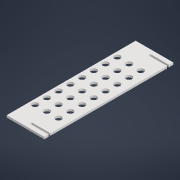
# Autodesk Inventor part: ChromoHolder
Saved by Autodesk Inventor 2021.3 (Build 253353000, 353)
## iProperties
Created: 2019-07-01
Part Number: ChromoHolder
Material: Generic
Document SubType Name: Modeling
Designer: eugen
Density: 1 g/cm^3
Appearance: Default
Author: eugen
Autodesk Inventor part; units mm, degrees
ref_plane "YZ Plane" through (0, 0, 0) normal (1, 0, 0) x (0, 1, 0)
ref_plane "XZ Plane" through (0, 0, 0) normal (0, 1, 0) x (-1, 0, 0)
ref_plane "XY Plane" through (0, 0, 0) normal (0, 0, 1) x (1, 0, 0)
sketch "Sketch1" plane through (0, 0, 0) normal (0, 1, 0) x (-1, 0, 0)
  line L0 (0, 0) -> (100.203, 0)
  line L1 (100.203, 0) -> (100.203, -387.1277)
  line L2 (100.203, -387.1277) -> (0, -387.1277)
  line L3 (0, -387.1277) -> (0, 0)
  line L4 (100.203, -63.0999) -> (100.203, -57.1309)
  line L5 (0, -12.7) -> (50.1015, -12.7)
  line L6 (51.3715, -13.97) -> (51.3715, -17.272)
  line L7 (50.1015, -18.542) -> (0, -18.542)
  line L8 (0, -18.542) -> (0, -12.7)
  line L9 (100.203, -374.4277) -> (100.203, -368.4587)
  line L10 (0, -374.4277) -> (50.1015, -374.4277)
  line L11 (51.3715, -373.1577) -> (51.3715, -369.8557)
  line L12 (50.1015, -368.5857) -> (0, -368.5857)
  line L13 (0, -368.5857) -> (0, -374.4277)
  circle A0 centre (50.1015, -70.1707) radius 9.1281
  line L14 (50.1015, 0) -> (50.1015, -387.1277) construction
  line L15 (14.8463, 0) -> (14.8463, -387.1277) construction
  circle A1 centre (50.1015, -105.4259) radius 9.1281
  circle A2 centre (50.1015, -140.6811) radius 9.1281
  circle A3 centre (50.1015, -175.9363) radius 9.1281
  circle A4 centre (50.1015, -211.1915) radius 9.1281
  circle A5 centre (50.1015, -246.4467) radius 9.1281
  circle A6 centre (50.1015, -281.7019) radius 9.1281
  circle A7 centre (50.1015, -316.9571) radius 9.1281
  circle A8 centre (14.8463, -70.1707) radius 9.1281
  circle A9 centre (14.8463, -105.4259) radius 9.1281
  circle A10 centre (14.8463, -140.6811) radius 9.1281
  circle A11 centre (14.8463, -175.9363) radius 9.1281
  circle A12 centre (14.8463, -211.1915) radius 9.1281
  circle A13 centre (14.8463, -246.4467) radius 9.1281
  circle A14 centre (14.8463, -281.7019) radius 9.1281
  circle A15 centre (14.8463, -316.9571) radius 9.1281
  line L16 (85.3567, -368.4587) -> (85.3567, -63.0999) construction
  circle A16 centre (85.3567, -70.1707) radius 9.1281
  circle A17 centre (85.3567, -105.4259) radius 9.1281
  circle A18 centre (85.3567, -140.6811) radius 9.1281
  circle A19 centre (85.3567, -175.9363) radius 9.1281
  circle A20 centre (85.3567, -211.1915) radius 9.1281
  circle A21 centre (85.3567, -246.4467) radius 9.1281
  circle A22 centre (85.3567, -281.7019) radius 9.1281
  circle A23 centre (85.3567, -316.9571) radius 9.1281
  line L17 (14.8463, -70.1707) -> (85.3567, -70.1707) construction
  arc A24 (50.1015, -374.4277) -> (51.3715, -373.1577) centre (50.1015, -373.1577) ccw
  arc A25 (51.3715, -369.8557) -> (50.1015, -368.5857) centre (50.1015, -369.8557) ccw
  arc A26 (50.1015, -18.542) -> (51.3715, -17.272) centre (50.1015, -17.272) ccw
  arc A27 (51.3715, -13.97) -> (50.1015, -12.7) centre (50.1015, -13.97) ccw
  point P0 (51.3715, -18.542)
  point P1 (51.3715, -12.7)
  point P2 (51.3715, -368.5857)
  point P3 (51.3715, -374.4277)
  point P4 (0, -18.542)
  point P5 (0, -368.5857)
  point P6 (94.2461, -248.5206)
  dimension "d10" = 35.2552
  dimension "d42" = 35.2552
  dimension "d0" = 100.203
  dimension "d1" = 387.1277
  dimension "d7" = 18.2563
  dimension "d11" = 35.2552
  dimension "d12" = 35.2552
  dimension "d13" = 35.2552
  dimension "d14" = 35.2552
  dimension "d15" = 35.2552
  dimension "d16" = 35.2552
  dimension "d17" = 35.2552
  dimension "d21" = 18.2563
  dimension "d22" = 35.2552
  dimension "d23" = 35.2552
  dimension "d24" = 35.2552
  dimension "d25" = 35.2552
  dimension "d26" = 35.2552
  dimension "d27" = 35.2552
  dimension "d28" = 35.2552
  dimension "d34" = 18.2563
  dimension "d35" = 35.2552
  dimension "d36" = 35.2552
  dimension "d37" = 35.2552
  dimension "d38" = 35.2552
  dimension "d39" = 35.2552
  dimension "d40" = 35.2552
  dimension "d41" = 35.2552
  dimension "d48" = 5.842
  dimension "d49" = 5.842
  dimension "d50" = 51.3715
  dimension "d51" = 12.7
  dimension "d52" = 12.7
  dimension "d53" = 175.9363
  dimension "d54" = 1.27
  constraints: 30 end point, 27 centre point, 23 equal radius, 14 point on line, 8 point on circle, 8 tangent, 6 horizontal, 6 parallel, 3 midpoint, 3 perpendicular, 1 collinear, 37 other
  measures "d0" distance of L1.end L2.end
  measures "d1" distance of L0.end L1.end
  measures "d7" diameter of A0
  measures "d11" distance of A1.centre A0.centre
  measures "d12" distance of A2.centre A1.centre
  measures "d13" distance of A3.centre A2.centre
  measures "d14" distance of A4.centre A3.centre
  measures "d15" distance of A4.centre A5.centre
  measures "d16" distance of A6.centre A5.centre
  measures "d17" distance of A6.centre A7.centre
  measures "d21" diameter of A8
  measures "d22" distance of A9.centre L17.start
  measures "d23" distance of A10.centre A9.centre
  measures "d24" distance of A11.centre A10.centre
  measures "d25" distance of A12.centre A11.centre
  measures "d26" distance of A12.centre A13.centre
  measures "d27" distance of A14.centre A13.centre
  measures "d28" distance of A14.centre A15.centre
  measures "d34" diameter of A16
  measures "d35" distance of A17.centre L17.end
  measures "d36" distance of A18.centre A17.centre
  measures "d37" distance of A19.centre A18.centre
  measures "d38" distance of A20.centre A19.centre
  measures "d39" distance of A20.centre point (85.357, -246.447)
  measures "d40" distance of A22.centre point (85.357, -246.447)
  measures "d41" distance of A22.centre A23.centre
  measures "d48" distance between parallel lines of L10 L12
  measures "d49" distance between parallel lines of L7 L5
  measures "d50" distance between parallel lines of L3 L6
  measures "d51" distance between parallel lines of L0 L5
  measures "d52" distance between parallel lines of L2 L10
  measures "d53" distance from line of L0 A11.centre
  measures "d54" radius of A24
extrude "Extrusion1" add sketch "Sketch1" along normal blind 6.35 contours L0 L1 L2 L3 L10 A24 L11 A25 L12 L7 A26 L6 A27 L5
equation "\"d10\" = d11"
equation "\"d42\" = d35"
equation "\"d12\" = d11"
equation "\"d13\" = d11"
equation "\"d14\" = d11"
equation "\"d15\" = d11"
equation "\"d16\" = d11"
equation "\"d17\" = d11"
equation "\"d22\" = d11"
equation "\"d23\" = d22"
equation "\"d24\" = d22"
equation "\"d25\" = d22"
equation "\"d26\" = d22"
equation "\"d27\" = d22"
equation "\"d28\" = d22"
equation "\"d36\" = d35"
equation "\"d37\" = d35"
equation "\"d38\" = d35"
equation "\"d39\" = d35"
equation "\"d40\" = d35"
equation "\"d41\" = d35"
body "Solid1"
